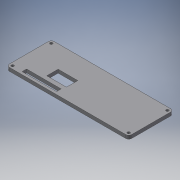
# Autodesk Inventor part: A8-0005
Saved by Autodesk Inventor 2016 SP2 (Build 200236200, 236)
## iProperties
Created: 2017-04-22
Part Number: A8-0005
Material: Generic
Document SubType Name: Modeling
Designer: EV
Density: 1 g/cm^3
Appearance: Default
Author: EV
Autodesk Inventor part; units mm, degrees
ref_plane "YZ Plane" through (0, 0, 0) normal (1, 0, 0) x (0, 1, 0)
ref_plane "XZ Plane" through (0, 0, 0) normal (0, 1, 0) x (-1, 0, 0)
ref_plane "XY Plane" through (0, 0, 0) normal (0, 0, 1) x (1, 0, 0)
sketch "Sketch1" plane through (0, 0, 0) normal (0, 1, 0) x (-1, 0, 0)
  line L0 (-4, 0) -> (-157, 0)
  line L1 (-161, -4) -> (-161, -55)
  line L2 (-157, -59) -> (-4, -59)
  line L3 (0, -55) -> (0, -4)
  line L4 (-17, -3.5) -> (-62.5, -3.5)
  line L5 (-62.5, -3.5) -> (-62.5, -9.5)
  line L6 (-62.5, -9.5) -> (-17, -9.5)
  line L7 (-17, -9.5) -> (-17, -3.5)
  line L8 (-38, -15) -> (-64, -15)
  line L9 (-64, -15) -> (-64, -30)
  line L10 (-64, -30) -> (-38, -30)
  line L11 (-38, -30) -> (-38, -15)
  arc A0 (0, -4) -> (-4, 0) centre (-4, -4) ccw
  arc A1 (-157, 0) -> (-161, -4) centre (-157, -4) ccw
  arc A2 (-161, -55) -> (-157, -59) centre (-157, -55) ccw
  arc A3 (-4, -59) -> (0, -55) centre (-4, -55) ccw
  point P0 (0, 0)
  point P1 (-161, 0)
  point P2 (0, -59)
  dimension "d0" = 161
  dimension "d1" = 59
  dimension "d2" = 6
  dimension "d3" = 45.5
  dimension "d4" = 26
  dimension "d5" = 15
  dimension "d6" = 3.5
  dimension "d7" = 15
  dimension "d8" = 17
  dimension "d9" = 38
  dimension "d10" = 4
  dimension "d20" = 51
  dimension "d21" = 153
  constraints: 24 end point, 8 point on circle, 8 tangent, 6 parallel, 6 point on line, 4 centre point, 3 equal radius, 3 horizontal, 3 perpendicular
  measures "d0" distance of point (0, 0) point (-161, 0)
  measures "d1" distance of point (0, -59) point (0, 0)
  measures "d2" distance of L4.end L5.end
  measures "d3" distance of L4.start L4.end
  measures "d4" distance of L8.start L8.end
  measures "d5" distance of L8.end L9.end
  measures "d6" distance between parallel lines of L0 L4
  measures "d7" distance between parallel lines of L0 L8
  measures "d8" distance between parallel lines of L3 L7
  measures "d9" distance between parallel lines of L3 L11
  measures "d10" radius of A0
  measures "d20" distance of A0.centre A3.centre
  measures "d21" distance of A1.centre A0.centre
extrude "Extrusion1" add sketch "Sketch1" along normal blind 4.5
sketch "Sketch2" plane through (0, 4.5, 0) normal (0, 1, 0) x (1, 0, 0)
  line L0 (38, 15) -> (38, 30) construction
  line L1 (38, 30) -> (64, 30) construction
  line L2 (64, 30) -> (64, 15) construction
  line L3 (64, 15) -> (38, 15) construction
  line L4 (17, 3.5) -> (17, 9.5) construction
  line L5 (17, 9.5) -> (62.5, 9.5) construction
  line L6 (62.5, 9.5) -> (62.5, 3.5) construction
  line L7 (62.5, 3.5) -> (17, 3.5) construction
  line L8 (4, 0) -> (157, 0) construction
  arc A0 (157, 0) -> (161, 4) centre (157, 4) ccw construction
  line L9 (161, 4) -> (161, 55) construction
  arc A1 (161, 55) -> (157, 59) centre (157, 55) ccw construction
  line L10 (157, 59) -> (4, 59) construction
  arc A2 (4, 59) -> (0, 55) centre (4, 55) ccw construction
  line L11 (0, 55) -> (0, 4) construction
  arc A3 (0, 4) -> (4, 0) centre (4, 4) ccw construction
  point P0 (0, 0)
  constraints: 4 coincident
hole "Hole1" at (4, 4.5, -55) at (4, 4.5, -4) at (157, 4.5, -4) at (157, 4.5, -55) direction (0, -1, 0) diameter 3.5 end through all
body "Solid1"
